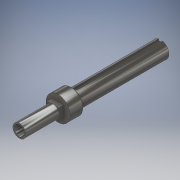
# Autodesk Inventor part: Adam's Motor Shaft Rev2
Saved by Autodesk Inventor 2019 (Build 230136000, 136)
## iProperties
Created: 2018-11-07
Part Number: Adam's Motor Shaft Rev2
Material: Steel, Alloy
Document SubType Name: Modeling
Designer: robinsat
Density: 7.73 g/cm^3
Appearance: Steel - Polished
Author: robinsat
Autodesk Inventor part; units mm, degrees
ref_plane "YZ Plane" through (0, 0, 0) normal (1, 0, 0) x (0, 1, 0)
ref_plane "XZ Plane" through (0, 0, 0) normal (0, 1, 0) x (-1, 0, 0)
sketch "Sketch1" plane through (0, 0, 0) normal (0, 0, 1) x (1, 0, 0)
  circle A0 centre (0, 0) radius 12.7
  dimension "d0" = 25.4
  constraints: 1 centre point, 1 coincident
  measures "d0" diameter of A0
extrude "Extrusion1" add sketch "Sketch1" along normal blind 155.575
sketch "Sketch2" plane through (0, 0, 155.575) normal (0, 0, 1) x (1, 0, 0)
  circle A0 centre (0, 0) radius 12.7 projected
  line L0 (-8.9803, 8.9803) -> (8.9803, 8.9803)
  line L1 (8.9803, 8.9803) -> (8.9803, -8.9803)
  line L2 (8.9803, -8.9803) -> (-8.9803, -8.9803)
  line L3 (-8.9803, -8.9803) -> (-8.9803, 8.9803)
  line L4 (-8.9803, 8.9803) -> (8.9803, -8.9803) construction
  line L5 (8.9803, 8.9803) -> (-8.9803, -8.9803) construction
  constraints: 12 end point, 2 midpoint, 2 parallel, 2 perpendicular, 1 horizontal, 1 point on circle
extrude "Extrusion2" add sketch "Sketch2" along normal blind 7.9375 contours L1 L2 L3 L0
sketch "Sketch3" plane through (0, 0, 163.5125) normal (0, 0, 1) x (1, 0, 0)
  circle A0 centre (0, 0) radius 9.9695
  dimension "d5" = 19.939
  constraints: 1 centre point, 1 coincident
  measures "d5" diameter of A0
extrude "Extrusion3" add sketch "Sketch3" along normal blind 50.8
sketch "Sketch4" plane through (0, 0, 214.3125) normal (0, 0, 1) x (1, 0, 0)
  circle A0 centre (0, 0) radius 7.9375
  dimension "d8" = 15.875
  constraints: 1 centre point, 1 coincident
  measures "d8" diameter of A0
extrude "Extrusion4" cut sketch "Sketch4" against normal up to surface (50.8 mm away)
sketch "Sketch5" plane through (0, 0, 0) normal (0, 0, -1) x (-1, 0, 0)
  line L0 (2.8575, 15.5575) -> (-2.8575, 15.5575)
  line L1 (-2.8575, 15.5575) -> (-2.8575, 9.8425)
  line L2 (-2.8575, 9.8425) -> (2.8575, 9.8425)
  line L3 (2.8575, 9.8425) -> (2.8575, 15.5575)
  arc A0 (8.9803, -8.9803) -> (8.9803, 8.9803) centre (0, 0) ccw projected
  line L4 (2.8575, 15.5575) -> (-2.8575, 9.8425) construction
  line L5 (-2.8575, 15.5575) -> (2.8575, 9.8425) construction
  point P0 (0, 12.7)
  point P1 (0, 12.7)
  dimension "d11" = 5.715
  constraints: 12 end point, 3 midpoint, 2 parallel, 2 perpendicular, 1 horizontal, 1 point on circle, 1 vertical alignment
  measures "d11" distance of L0.start L0.end
extrude "Extrusion5" cut sketch "Sketch5" against normal blind 129.8575
fillet "Fillet2" radius 2.8575 2 edges at (-2.8575, 11.1084, 129.8575) (2.8575, 11.1084, 129.8575)
sketch "Sketch6" plane through (0, 0, 155.575) normal (0, 0, 1) x (1, 0, 0)
  circle A0 centre (0, 0) radius 18.415
  dimension "d16" = 36.83
  constraints: 1 centre point, 1 coincident
  measures "d16" diameter of A0
ref_plane "Work Plane1" through (0, 12.7, 129.8575) normal (0, 0, 1) x (1, 0, 0)
sketch "Sketch7" plane through (0, 12.7, 129.8575) normal (0, 0, 1) x (1, 0, 0)
  circle A0 centre (0, -12.7) radius 7.9375 projected
  circle A1 centre (0, -12.7) radius 14.097
  constraints: 1 centre point, 1 coincident
extrude "Extrusion6" add sketch "Sketch6" against normal blind 19.05
fillet "Fillet3" radius 4.7625 1 edges at (-12.7, 0, 136.525)
body "Solid1"
